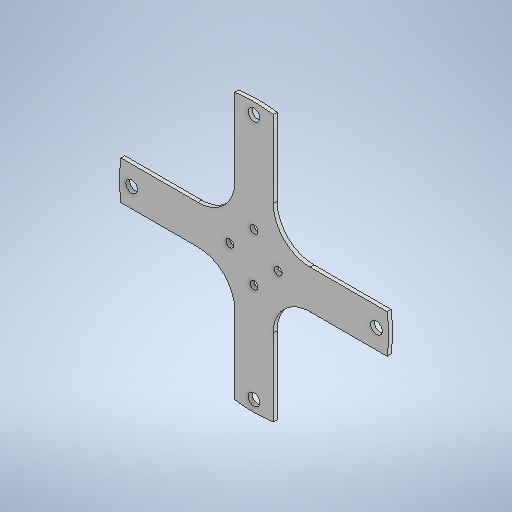
# Autodesk Inventor part: steering sheet
Saved by Autodesk Inventor 2025 (Build 290162000, 162)
## iProperties
Created: 2025-01-07
Part Number: steering sheet
Material: Generic
Document SubType Name: Modeling
Designer: 5014070
Density: 1 g/cm^3
Appearance: Default
Author: 5014070
Autodesk Inventor part; units mm, degrees
ref_plane "YZ Plane" through (0, 0, 0) normal (1, 0, 0) x (0, 1, 0)
ref_plane "XZ Plane" through (0, 0, 0) normal (0, 1, 0) x (-1, 0, 0)
ref_plane "XY Plane" through (0, 0, 0) normal (0, 0, 1) x (1, 0, 0)
sketch "Sketch1" plane through (0, 0, 0) normal (0, 0, 1) x (1, 0, 0)
  line L0 (-60.8901, 2.539) -> (2.3555, 66.2618)
  line L1 (2.3555, 66.2618) -> (65.601, 2.539)
  line L2 (65.601, 2.539) -> (2.3555, -61.1838)
  line L3 (2.3555, -61.1838) -> (-60.8901, 2.539)
  circle A0 centre (2.3555, 66.2618) radius 3
  circle A1 centre (-60.8901, 2.539) radius 3
  circle A2 centre (2.3555, -61.1838) radius 3
  circle A3 centre (65.601, 2.539) radius 3
  line L4 (-2.6445, 61.2618) -> (7.3555, 71.2618) construction
  line L5 (7.3555, 61.2618) -> (-2.6445, 71.2618) construction
  line L6 (-65.8901, -2.461) -> (-55.8901, 7.539) construction
  line L7 (-55.8901, -2.461) -> (-65.8901, 7.539) construction
  circle A4 centre (2.3555, 2.539) radius 100
  circle A5 centre (2.3555, 2.539) radius 70
  line L8 (65.601, 2.539) -> (-60.889, 2.539)
  line L9 (-70.889, -7.461) -> (-70.889, 12.539)
  line L10 (-70.889, 12.539) -> (-50.889, 12.539)
  line L11 (-50.889, 12.539) -> (-50.889, -7.461)
  line L12 (-50.889, -7.461) -> (-70.889, -7.461)
  line L13 (-70.889, -7.461) -> (-50.889, 12.539) construction
  line L14 (-70.889, 12.539) -> (-50.889, -7.461) construction
  line L15 (55.601, -7.461) -> (55.601, 12.539)
  line L16 (55.601, 12.539) -> (75.601, 12.539)
  line L17 (75.601, 12.539) -> (75.601, -7.461)
  line L18 (75.601, -7.461) -> (55.601, -7.461)
  line L19 (55.601, -7.461) -> (75.601, 12.539) construction
  line L20 (55.601, 12.539) -> (75.601, -7.461) construction
  line L21 (2.3555, 66.2618) -> (2.3555, 56.2618)
  line L22 (2.3555, 56.2618) -> (-7.5696, 56.2618)
  line L23 (-7.5696, 56.2618) -> (-7.5696, 71.8318)
  line L24 (2.3555, 56.2618) -> (12.2806, 56.2618)
  line L25 (12.2806, 56.2618) -> (12.2806, 71.8318)
  line L26 (2.3555, -61.1838) -> (2.3555, -51.1838)
  line L27 (2.3555, -51.1838) -> (-7.5696, -51.1838)
  line L28 (-7.5696, -66.7538) -> (-7.5696, -51.1838)
  line L29 (2.3555, -51.1838) -> (12.2806, -51.1838)
  line L30 (12.2806, -51.1838) -> (12.2806, -66.7538)
  line L31 (-50.965, 12.539) -> (55.601, 12.539)
  line L32 (55.601, 12.539) -> (55.601, -7.461)
  line L33 (55.601, -7.461) -> (-50.965, -7.461)
  line L34 (-50.965, -7.461) -> (-50.965, 12.539)
  line L35 (12.2806, -51.1838) -> (-7.5696, -51.1838)
  line L36 (-7.5696, -51.1838) -> (-7.5696, 56.2618)
  line L37 (-7.5696, 56.2618) -> (12.2806, 56.2618)
  line L38 (12.2806, 56.2618) -> (12.2806, -51.1838)
  circle A6 centre (2.3555, 2.539) radius 69.5
  circle A7 centre (2.3555, 2.539) radius 7
  line L39 (2.3555, 2.539) -> (14.8555, 2.539)
  circle A8 centre (14.8555, 2.539) radius 2
  circle A9 centre (2.3555, 15.039) radius 2
  circle A10 centre (-10.1445, 2.539) radius 2
  circle A11 centre (2.3555, -9.961) radius 2
  point P0 (0, 0)
  point P1 (-60.8901, 2.539)
  point P2 (-66.9266, 12.539)
  point P3 (-66.9266, -7.461)
  point P4 (-50.965, -7.461)
  point P5 (12.2806, 12.539)
  point P6 (-7.5696, 12.539)
  point P7 (-50.889, -7.461)
  point P8 (-7.5696, -7.461)
  point P9 (12.2806, -7.461)
  point P10 (71.6375, -7.461)
  point P11 (71.6375, 12.539)
  point P12 (12.2806, 71.3266)
  point P13 (-7.5696, 71.3266)
  point P14 (-7.5696, -66.2487)
  point P15 (12.2806, -66.2487)
  point P16 (71.1323, -7.461)
  point P17 (71.1323, 12.539)
  point P18 (-66.4214, 12.539)
  point P19 (-66.4214, -7.461)
  dimension "d0" = 6
  dimension "d1" = 6
  dimension "d2" = 6
  dimension "d3" = 6
  dimension "d8" = 200
  dimension "d9" = 140
  dimension "d10" = 126.49
  dimension "d11" = 20
  dimension "d12" = 20
  dimension "d13" = 20
  dimension "d14" = 20
  dimension "d18" = 10
  dimension "d19" = 10
  dimension "d22" = 139
  dimension "d24" = 14
  dimension "d25" = 12.5
  dimension "d26" = 4
  dimension "d29" = 360
  constraints: 80 end point, 14 point on line, 12 centre point, 10 parallel, 8 coincident, 8 midpoint, 7 perpendicular, 4 point on circle, 3 horizontal, 2 vertical, 9 other
  measures "d0" diameter of A0
  measures "d1" diameter of A1
  measures "d2" diameter of A2
  measures "d3" diameter of A3
  measures "d8" diameter of A4
  measures "d9" diameter of A5
  measures "d10" distance of L8.start L8.end
  measures "d11" distance of L9.start L9.end
  measures "d12" distance of L9.end L10.end
  measures "d13" distance of L15.start L15.end
  measures "d14" distance of L15.end L16.end
  measures "d18" distance of L21.start L21.end
  measures "d19" distance of L26.start L26.end
  measures "d22" diameter of A6
  measures "d24" diameter of A7
  measures "d25" distance of L39.start L39.end
  measures "d26" diameter of A8
extrude "Extrusion1" add sketch "Sketch1" along normal blind 2 contours L34 L8 A1 L0 | L0 A1 L3 L12 A6 L10 | L10 L11 L8 L34 | L23 A6 L25 L1 A0 L0 | L0 A0 L21 L22 | L22 L24 L38 L31 L36 | L31 L36 L8 A10 L11 | L34 L3 A1 L8 | L8 L11 L12 L34 | L21 A0 L1 L24 | L31 L38 L8 A7 L36 | L8 A10 L36 L33 L11 | L31 L15 L8 A8 L38 | L8 A7 L38 L33 L36 | L28 L3 A2 L2 L30 A6 | L27 L26 A2 L3 | L36 L33 L38 L29 L27 | L16 A6 L18 L2 A3 L1 | L1 A3 L8 L15 L16 | L8 A8 L15 L33 L38 | A7 L8 | L8 A7 | L29 L2 A2 L26 | L8 A3 L2 L18 L15
fillet "Fillet1" radius 19.05 4 edges at (12.2806, 12.539, 1) (-7.5696, 12.539, 1) (-7.5696, -7.461, 1) (12.2806, -7.461, 1)
body "Solid1"
